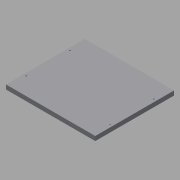
# Autodesk Inventor part: ed30 panel solar
Saved by Autodesk Inventor 2014 (Build 180170000, 170)
## iProperties
Created: 2016-10-24
Part Number: ed30 panel solar
Material: Polycarbonate, Smoke
Document SubType Name: Modeling
Designer: Cristian
Density: 1 g/cm^3
Appearance: Polycarbonate - Smoked
Author: Cristian
Autodesk Inventor part; units mm, degrees
ref_plane "YZ Plane" through (0, 0, 0) normal (1, 0, 0) x (0, 1, 0)
ref_plane "XZ Plane" through (0, 0, 0) normal (0, 1, 0) x (-1, 0, 0)
ref_plane "XY Plane" through (0, 0, 0) normal (0, 0, 1) x (1, 0, 0)
sketch "Sketch1" plane through (0, 0, 0) normal (0, 0, 1) x (1, 0, 0)
  line L0 (-255, -225) -> (255, -225)
  line L1 (255, -225) -> (255, 225)
  line L2 (255, 225) -> (-255, 225)
  line L3 (-255, 225) -> (-255, -225)
  line L4 (-255, -225) -> (255, 225) construction
  line L5 (255, -225) -> (-255, 225) construction
  point P0 (0, 0)
  dimension "d0" = 510
  dimension "d1" = 450
  constraints: 12 end point, 2 midpoint, 2 parallel, 1 horizontal, 1 perpendicular
  measures "d0" distance of L2.end L1.end
  measures "d1" distance of L1.end L0.end
extrude "Extrusion1" add sketch "Sketch1" along normal blind 25
sketch "Sketch2" plane through (0, 0, 25) normal (0, 0, 1) x (1, 0, 0)
  line L0 (-255, -225) -> (255, -225) construction
  line L1 (255, -225) -> (255, 225) construction
  line L2 (255, 225) -> (-255, 225) construction
  line L3 (-255, 225) -> (-255, -225) construction
  line L4 (255, 225) -> (255, 125) construction
  line L5 (255, -225) -> (255, -125) construction
  line L6 (255, 125) -> (-255, 125) construction
  line L7 (255, -125) -> (-255, -125) construction
  line L8 (0, -125) -> (239.5, -125) construction
  line L9 (0, -125) -> (-239.5, -125) construction
  circle A0 centre (-239.5, -125) radius 3.5
  circle A1 centre (239.5, -125) radius 3.5
  line L10 (0, 125) -> (239.5, 125) construction
  line L11 (0, 125) -> (-239.5, 125) construction
  circle A2 centre (-239.5, 125) radius 3.5
  circle A3 centre (239.5, 125) radius 3.5
  point P0 (0, 0)
  dimension "d4" = 100
  dimension "d5" = 100
  dimension "d6" = 239.5
  dimension "d7" = 239.5
  dimension "d8" = 7
  dimension "d9" = 7
  dimension "d10" = 239.5
  dimension "d11" = 239.5
  dimension "d12" = 7
  dimension "d13" = 7
  constraints: 16 end point, 8 point on line, 4 centre point, 4 coincident, 2 horizontal, 2 midpoint
  measures "d4" distance of L1.end L4.end
  measures "d5" distance of L0.end L5.end
  measures "d6" distance of L8.start L8.end
  measures "d7" distance of L8.start L9.end
  measures "d8" diameter of A0
  measures "d9" diameter of A1
  measures "d10" distance of L10.start L10.end
  measures "d11" distance of L10.start L11.end
  measures "d12" diameter of A2
  measures "d13" diameter of A3
extrude "Extrusion2" cut sketch "Sketch2" against normal blind 11
body "Solid1"
